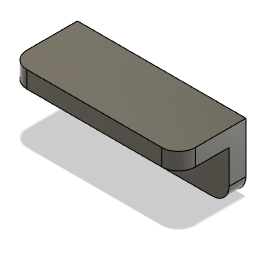
Trigger Support (Autodesk Fusion 360 design; units mm, degrees)
Autodesk Fusion 360 part; units mm, degrees
sketch "Sketch1" plane through (0, 0, 0) normal (0, 0, 1) x (1, 0, 0)
  line L0 (-16.0699, 13.472) -> (-6.0699, 13.472)
  line L1 (-6.0699, 13.472) -> (-6.0699, 9.472)
  line L2 (-6.0699, 9.472) -> (-16.0699, 9.472)
  line L3 (-16.0699, 9.472) -> (-16.0699, 13.472)
  dimension "d1" = 10
  dimension "d2" = 4
  constraint horizontal L0
  constraint vertical L1
  constraint horizontal L2
  constraint vertical L3
  measures "d1" distance of L0.start L0.end
  measures "d2" distance of L0.start L2.end
extrude "Extrude1" add sketch "Sketch1" along normal blind 1
sketch "Sketch2" plane through (0, 0, 1) normal (0, 0, 1) x (1, 0, 0)
  line L0 (-16.0699, 9.472) -> (-6.0699, 9.472)
  line L1 (-6.0699, 9.472) -> (-6.0699, 13.472)
  line L2 (-6.0699, 13.472) -> (-16.0699, 13.472)
  line L3 (-16.0699, 13.472) -> (-16.0699, 9.472)
  line L4 (-16.0699, 13.472) -> (-6.0699, 13.472)
  line L5 (-6.0699, 13.472) -> (-6.0699, 12.472)
  line L6 (-6.0699, 12.472) -> (-16.0699, 12.472)
  line L7 (-16.0699, 12.472) -> (-16.0699, 13.472)
  dimension "d5" = 1
  dimension "d6" = 10
  constraint horizontal L4
  constraint vertical L5
  constraint horizontal L6
  constraint vertical L7
  constraint coincident L2.end L3.start
  measures "d5" distance of L2.end L6.end
  measures "d6" distance of L2.end L1.end
extrude "Extrude2" add sketch "Sketch2" along normal blind 3 contours L1 L2 L3 L4 L5 L6 L7
fillet "Fillet1" radius 1 1 edges at (-6.0699, 9.472, 0.5)
fillet "Fillet2" radius 1 1 edges at (-16.0699, 9.472, 0.5)
fillet "Fillet3" radius 1 1 edges at (-16.0699, 12.972, 4)
fillet "Fillet4" radius 1 1 edges at (-6.0699, 12.972, 4)
